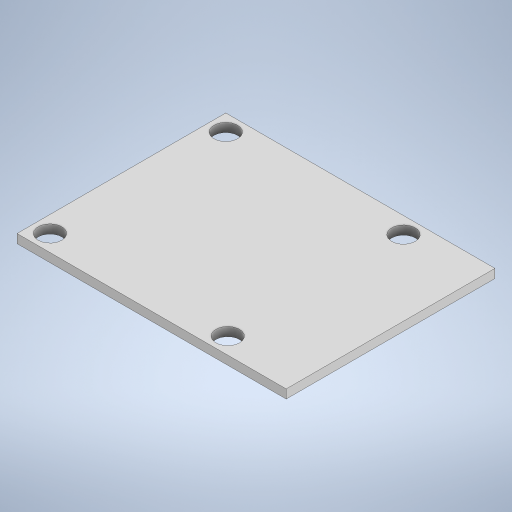
# Autodesk Inventor part: _Reference_PCB
Saved by Autodesk Inventor 2023.2 (Build 272271000, 271)
## iProperties
Created: 2023-02-13
Part Number: _Reference_PCB
Material: Generic
Document SubType Name: Modeling
Designer: atrus
Density: 1 g/cm^3
Appearance: Default
Author: atrus
Autodesk Inventor part; units mm, degrees
ref_plane "YZ Plane" through (0, 0, 0) normal (1, 0, 0) x (0, 1, 0)
ref_plane "XZ Plane" through (0, 0, 0) normal (0, 1, 0) x (-1, 0, 0)
ref_plane "XY Plane" through (0, 0, 0) normal (0, 0, 1) x (1, 0, 0)
sketch "Sketch1" plane through (0, 0, 0) normal (0, 1, 0) x (-1, 0, 0)
  line L0 (49, 0) -> (0, 0)
  line L1 (0, 0) -> (0, -38)
  line L2 (0, -38) -> (49, -38)
  line L3 (49, -38) -> (49, 0)
  dimension "d0" = 38
  dimension "d1" = 49
  constraints: 8 end point, 2 parallel, 1 coincident, 1 horizontal, 1 perpendicular
  measures "d0" distance of L0.end L1.end
  measures "d1" distance of L1.end L2.end
extrude "Extrusion1" add sketch "Sketch1" along normal blind 1.6
sketch "Sketch2" plane through (0, 1.6, 0) normal (0, 1, 0) x (1, 0, 0)
  line L0 (-49, 38) -> (-49, 0) construction
  line L1 (-49, 19) -> (0, 19) construction
  line L2 (0, 0) -> (0, 38) construction
  line L3 (0, 38) -> (-49, 38) projected
  point P0 (-13.65, 3)
  point P1 (-13.65, 35)
  point P2 (-46, 35)
  point P3 (-46, 3)
  dimension "d5" = 32.35
  dimension "d6" = 3
  dimension "d14" = 3
  constraints: 2 end point, 2 horizontal alignment, 2 midpoint, 1 symmetric about line, 1 vertical alignment
  measures "d5" distance of point (-13.65, 35) point (-46, 35)
  measures "d6" distance from line of L0 point (-46, 35)
  measures "d14" distance from line of L3 point (-46, 35)
hole "Hole1" at (-13.65, 1.6, -3) at (-13.65, 1.6, -35) at (-46, 1.6, -35) at (-46, 1.6, -3) direction (0, -1, 0) diameter 4.305 end through all clearance for "Flat Head Machine Screw (82)" size "#6" standard "Ansi Unified Screw Threads"
body "Solid1"
